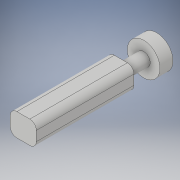
# Autodesk Inventor part: car suspension wheel joint
Saved by Autodesk Inventor 2019 (Build 230136000, 136)
## iProperties
Created: 2019-03-16
Part Number: car suspension wheel joint
Material: Generic
Document SubType Name: Modeling
Designer: Manoj
Density: 1 g/cm^3
Appearance: Default
Author: Manoj
Autodesk Inventor part; units mm, degrees
ref_plane "YZ Plane" through (0, 0, 0) normal (1, 0, 0) x (0, 1, 0)
ref_plane "XZ Plane" through (0, 0, 0) normal (0, 1, 0) x (-1, 0, 0)
ref_plane "XY Plane" through (0, 0, 0) normal (0, 0, 1) x (1, 0, 0)
sketch "Sketch1" plane through (0, 0, 0) normal (0, 1, 0) x (-1, 0, 0)
  line L0 (200, 750) -> (-200, 750)
  line L1 (-200, 750) -> (-200, -750)
  line L2 (-200, -750) -> (200, -750)
  line L3 (200, -750) -> (200, 750)
  line L4 (200, 0) -> (-200, 0) construction
  line L5 (0, -750) -> (0, 750) construction
  point P0 (0, 0)
  point P1 (0, 0)
  dimension "d0" = 1500
  dimension "d1" = 400
  constraints: 12 end point, 5 midpoint, 2 parallel, 1 coincident, 1 horizontal, 1 perpendicular
  measures "d0" distance of L2.end L0.start
  measures "d1" distance of L1.end L2.end
extrude "Extrusion1" add sketch "Sketch1" along normal blind 350
sketch "Sketch2" plane through (200, 0, -750) normal (0, 0, -1) x (-1, 0, 0)
  line L0 (200, 0) -> (200, 350) construction
  line L1 (400, 350) -> (0, 350) construction
  line L2 (400, 0) -> (400, 350) construction
  line L3 (400, 175) -> (0, 175) construction
  line L4 (0, 0) -> (0, 350) construction
  circle A0 centre (200, 175) radius 100
  dimension "d4" = 200
  constraints: 4 end point, 4 midpoint, 1 centre point
  measures "d4" diameter of A0
extrude "Extrusion2" add sketch "Sketch2" along normal blind 350
sketch "Sketch3" plane through (0, 175, -1100) normal (0, 0, -1) x (-1, 0, 0)
  line L0 (-200, 175) -> (200, 175) construction
  line L1 (0, 175) -> (0, -175) construction
  circle A0 centre (0, 0) radius 100 construction
  circle A1 centre (0, 0) radius 250
  dimension "d7" = 500
  constraints: 2 end point, 1 centre point, 1 coincident, 1 midpoint, 1 vertical
  measures "d7" diameter of A1
extrude "Extrusion3" add sketch "Sketch3" along normal blind 200
fillet "Fillet1" radius 100 4 edges at (200, 350, 0) (-200, 350, 0) (200, 0, 0) (-200, 0, 0)
body "Solid1"
